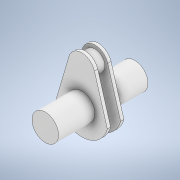
# Autodesk Inventor part: Crank_Shaft
Saved by Autodesk Inventor 2021 (Build 250183000, 183)
## iProperties
Created: 2021-04-09
Part Number: Crank_Shaft
Material: Stainless Steel
Document SubType Name: Modeling
Designer: tommy
Density: 8 g/cm^3
Appearance: Smooth - White
Author: tommy
Autodesk Inventor part; units mm, degrees
ref_plane "YZ Plane" through (0, 0, 0) normal (1, 0, 0) x (0, 1, 0)
ref_plane "XZ Plane" through (0, 0, 0) normal (0, 1, 0) x (-1, 0, 0)
ref_plane "XY Plane" through (0, 0, 0) normal (0, 0, 1) x (1, 0, 0)
sketch "Sketch1" plane through (0, 0, 0) normal (0, 0, 1) x (1, 0, 0)
  circle A0 centre (0, 0) radius 19.05
  circle A1 centre (0, 63.5) radius 19.05
  line L0 (0, -78.74) -> (0, 116.84) construction
  circle A2 centre (0, 63.5) radius 25.4
  circle A3 centre (0, 0) radius 25.4
  arc A4 (-49.069, -13.148) -> (49.069, -13.148) centre (0, 0) ccw
  line L1 (0, 0) -> (49.069, -13.148) construction
  line L2 (0, 0) -> (50.8, 0) construction
  line L3 (0, 0) -> (-49.069, -13.148) construction
  line L4 (-49.069, -13.148) -> (-24.364, 70.6803)
  line L5 (49.069, -13.148) -> (24.364, 70.6803)
  dimension "crank_dia" = 38.1
  dimension "d2" = 38.1
  dimension "crank_ctc" = 63.5
  dimension "crank_wt" = 6.35
  dimension "d8" = 6.35
  dimension "crank_rad" = 50.8
  dimension "d10" = 15
  dimension "d13" = 150
  constraints: 10 end point, 5 centre point, 4 point on circle, 3 coincident, 2 tangent, 1 equal length, 1 horizontal, 1 point on line
  measures "crank_dia" diameter of A0
  measures "d2" diameter of A1
  measures "crank_ctc" distance of A1.centre point (0, 0)
  measures "crank_wt" radial gap between concentric circles of A2 A1
  measures "d8" radial gap between concentric circles of A3 A0
  measures "crank_rad" radius of A4
  measures "d10" angle of L1 L2
  measures "d13" angle of L3 L1
extrude "Extrusion1" add sketch "Sketch1" along normal blind 9.525 contours A1
extrude "Extrusion2" add sketch "Sketch1" along normal blind 6.35 from surface at 9.525 contours A1 | A2 | A2 L5 A4 L4
extrude "Extrusion3" add sketch "Sketch1" along normal blind 76.2 from surface at 9.525 contours A0 | A3
mirror "Mirror1" about plane through (0, 0, 0) normal (0, 0, 1) of "Extrusion1", "Extrusion2", "Extrusion3"
equation "\"d2\" = 2 * pin_dia"
equation "\"d8\" = crank_wt"
equation "\"pin_dia\" = 19.05"
body "Solid1"
